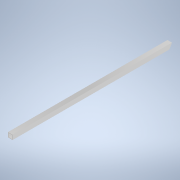
# Autodesk Inventor part: aluminumBallHandlerHypotenuse
Saved by Autodesk Inventor 2020.2 (Build 242310000, 310)
## iProperties
Created: 2020-01-16
Part Number: aluminumBallHandlerHypotenuse
Material: Aluminum 6061-AHC
Document SubType Name: Modeling
Designer: robst
Density: 2.7 g/cm^3
Appearance: Aluminum - Dark
Author: robst
Autodesk Inventor part; units mm, degrees
ref_plane "YZ Plane" through (0, 0, 0) normal (1, 0, 0) x (0, 1, 0)
ref_plane "XZ Plane" through (0, 0, 0) normal (0, 1, 0) x (-1, 0, 0)
ref_plane "XY Plane" through (0, 0, 0) normal (0, 0, 1) x (1, 0, 0)
sketch "Sketch2" plane through (0, 0, 0) normal (0, 0, 1) x (1, 0, 0)
  line L0 (-12.7, -12.7) -> (12.7, -12.7)
  line L1 (12.7, -12.7) -> (12.7, 12.7)
  line L2 (12.7, 12.7) -> (-12.7, 12.7)
  line L3 (-12.7, 12.7) -> (-12.7, -12.7)
  line L4 (-12.7, -12.7) -> (12.7, 12.7) construction
  line L5 (12.7, -12.7) -> (-12.7, 12.7) construction
  line L6 (-9.525, -9.525) -> (9.525, -9.525)
  line L7 (9.525, -9.525) -> (9.525, 9.525)
  line L8 (9.525, 9.525) -> (-9.525, 9.525)
  line L9 (-9.525, 9.525) -> (-9.525, -9.525)
  line L10 (-9.525, -9.525) -> (9.525, 9.525) construction
  line L11 (9.525, -9.525) -> (-9.525, 9.525) construction
  point P0 (0, 0)
  dimension "d0" = 25.4
  dimension "d1" = 25.4
  dimension "d2" = 3.175
  dimension "d3" = 3.175
  constraints: 24 end point, 5 parallel, 4 midpoint, 2 perpendicular, 1 horizontal
  measures "d0" distance of L0.start L0.end
  measures "d1" distance of L1.end L0.end
  measures "d2" distance between parallel lines of L6 L0
  measures "d3" distance between parallel lines of L9 L3
extrude "Extrusion1" add sketch "Sketch2" along normal mid plane 879.856
sketch "Sketch3" plane through (12.7, -12.7, 439.928) normal (1, 0, 0) x (0, 0, -1)
  line L0 (879.856, 25.4) -> (879.856, 0) projected
  line L1 (879.856, 25.4) -> (865.1913, 0)
  line L2 (879.856, 0) -> (0, 0) projected
  line L3 (865.1913, 0) -> (879.856, 0)
  line L4 (879.856, 25.4) -> (0, 25.4) projected
  line L5 (879.856, 0) -> (879.856, 25.4)
  point P0 (439.928, 12.7)
  dimension "d6" = 30
  constraints: 6 end point, 1 collinear, 1 point on line, 1 vertical
  measures "d6" angle of L1 L0
extrude "Extrusion2" cut sketch "Sketch3" against normal through all
sketch "Sketch4" plane through (12.7, -12.7, 439.928) normal (1, 0, 0) x (0, 0, -1)
  line L0 (0, 25.4) -> (0, 0) projected
  line L1 (0, 25.4) -> (36.2286, 4.4834)
  line L2 (36.2286, 4.4834) -> (43.9941, 0)
  line L3 (865.1913, 0) -> (0, 0) projected
  line L4 (0, 25.4) -> (0, 0)
  line L5 (0, 0) -> (43.9941, 0)
  point P0 (439.928, 12.7)
  dimension "d9" = 60
  constraints: 8 end point, 2 point on line, 1 collinear, 1 vertical
  measures "d9" angle of L1 L0
extrude "Extrusion3" cut sketch "Sketch4" against normal through all
body "Solid1"
